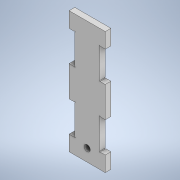
# Autodesk Inventor part: rail
Saved by Autodesk Inventor 2020 (Build 240168000, 168)
## iProperties
Created: 2019-12-19
Part Number: rail
Material: Générique
Document SubType Name: Modeling
Designer: damien
Density: 1 g/cm^3
Appearance: Par défaut
Author: damien
Autodesk Inventor part; units mm, degrees
ref_plane "YZ Plane" through (0, 0, 0) normal (1, 0, 0) x (0, 1, 0)
ref_plane "XZ Plane" through (0, 0, 0) normal (0, 1, 0) x (-1, 0, 0)
ref_plane "XY Plane" through (0, 0, 0) normal (0, 0, 1) x (1, 0, 0)
sketch "Esquisse1" plane through (0, 0, 0) normal (0, 0, 1) x (1, 0, 0)
  line L0 (0, 0) -> (-118.5, 0)
  line L1 (-118.5, 0) -> (-118.5, -400)
  line L2 (-118.5, -400) -> (0, -400)
  line L3 (0, -400) -> (0, 0)
  dimension "d0" = 400
  dimension "d3" = 118.5
  constraints: 8 end point, 3 perpendicular, 1 horizontal
  measures "d0" distance of L0.end L1.end
  measures "d3" distance of L0.start L0.end
extrude "Extrusion1" add sketch "Esquisse1" along normal blind 18.55
sketch "Esquisse2" plane through (0, 0, 18.55) normal (0, 0, 1) x (1, 0, 0)
  line L0 (-118.5, 0) -> (-118.5, -400) construction
  line L1 (-118.5, -50) -> (-99.95, -50)
  line L2 (-99.95, -50) -> (-99.95, -150)
  line L3 (-99.95, -150) -> (-118.5, -150)
  line L4 (-118.5, -150) -> (-118.5, -50)
  line L5 (-118.5, -250) -> (-99.95, -250)
  line L6 (-99.95, -250) -> (-99.95, -350)
  line L7 (-99.95, -350) -> (-118.5, -350)
  line L8 (-118.5, -350) -> (-118.5, -250)
  line L9 (0, 0) -> (-118.5, 0) projected
  line L10 (-118.5, -400) -> (0, -400) projected
  line L11 (-59.25, 0) -> (-59.25, -400) construction
  line L12 (0, 0) -> (0, -400) construction
  line L13 (0, -50) -> (-18.55, -50)
  line L14 (-18.55, -50) -> (-18.55, -150)
  line L15 (-18.55, -150) -> (0, -150)
  line L16 (0, -150) -> (0, -50)
  line L17 (0, -250) -> (-18.55, -250)
  line L18 (-18.55, -250) -> (-18.55, -350)
  line L19 (-18.55, -350) -> (0, -350)
  line L20 (0, -350) -> (0, -250)
  dimension "d27" = 18.55
  dimension "d28" = 100
  dimension "d29" = 100
  dimension "d30" = 100
  dimension "d31" = 50
  dimension "d32" = 50
  constraints: 36 end point, 8 symmetric about line, 4 parallel, 4 point on line, 2 horizontal, 2 midpoint, 2 perpendicular, 1 collinear
  measures "d27" distance of L2.end L3.end
  measures "d28" distance of L1.end L2.end
  measures "d29" distance of L5.end L6.end
  measures "d30" distance between parallel lines of L5 L3
  measures "d31" distance between parallel lines of L9 L1
  measures "d32" distance between parallel lines of L10 L7
extrude "Extrusion2" cut sketch "Esquisse2" against normal blind 18.55
sketch "Esquisse3" plane through (0, 0, 18.55) normal (0, 0, 1) x (1, 0, 0)
  circle A0 centre (-59, -360) radius 10
  line L0 (0, -400) -> (0, 0) projected
  line L1 (-118.5, -400) -> (0, -400) projected
  line L2 (-118.5, -350) -> (-118.5, -400) projected
  dimension "d21" = 59
  dimension "d22" = 20
  dimension "d23" = 40
  dimension "d33" = 59.5
  constraints: 1 centre point
  measures "d21" distance from line of L0 A0.centre
  measures "d22" diameter of A0
  measures "d23" distance from line of L1 A0.centre
  measures "d33" distance from line of L2 A0.centre
extrude "Extrusion3" cut sketch "Esquisse3" against normal blind 18.55
sketch "Esquisse4" plane through (0, 0, 18.55) normal (0, 0, 1) x (1, 0, 0)
  line L0 (-99.95, -50) -> (-99.95, -150) projected
  circle A0 centre (-99.95, -50) radius 1.5875
  circle A1 centre (-18.55, -50) radius 1.5875
  circle A2 centre (-99.95, -150) radius 1.5875
  line L1 (-18.55, -150) -> (0, -150) projected
  circle A3 centre (-18.55, -150) radius 1.5875
  circle A4 centre (-99.95, -250) radius 1.5875
  circle A5 centre (-18.55, -250) radius 1.5875
  line L2 (-99.95, -350) -> (-99.95, -250) projected
  circle A6 centre (-99.95, -350) radius 1.5875
  line L3 (-18.55, -250) -> (-18.55, -350) projected
  circle A7 centre (-18.55, -350) radius 1.5875
  point P0 (0, 0)
  dimension "d34" = 3.175
  constraints: 8 centre point, 7 equal radius, 3 coincident
  measures "d34" diameter of A0
extrude "Extrusion4" cut sketch "Esquisse4" against normal blind 18.55
